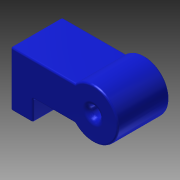
# Autodesk Inventor part: Lego Leg
Saved by Autodesk Inventor 2013 (Build 170138000, 138)
## iProperties
Created: 2013-09-06
Part Number: Lego Leg
Material: Generic
Document SubType Name: Modeling
Designer: 200395375
Density: 1 g/cm^3
Mass: 0.53052 g
Surface Area: 7.06359 cm^2
Volume: 0.53052 cm^3
Author: 200395375
Autodesk Inventor part; units mm, degrees
ref_plane "YZ Plane" through (0, 0, 0) normal (1, 0, 0) x (0, 1, 0)
ref_plane "XZ Plane" through (0, 0, 0) normal (0, 1, 0) x (-1, 0, 0)
ref_plane "XY Plane" through (0, 0, 0) normal (0, 0, 1) x (1, 0, 0)
sketch "Sketch1" plane through (0, 0, 0) normal (0, 1, 0) x (-1, 0, 0)
  line L0 (0, 0) -> (8.18, 0)
  line L1 (8.18, 0) -> (8.18, -7.83)
  line L2 (8.18, -7.83) -> (5.01, -7.83)
  line L3 (5.01, -7.83) -> (5.01, -4.86)
  line L4 (5.01, -4.86) -> (0, -4.86)
  line L5 (0, -4.86) -> (0, 0)
  dimension "d0" = 8.18
  dimension "d1" = 7.83
  dimension "d2" = 3.17
  dimension "d3" = 2.97
  constraints: 12 end point, 3 parallel, 2 perpendicular, 1 horizontal
  measures "d0" distance of L0.start L0.end
  measures "d1" distance of L0.end L1.end
  measures "d2" distance of L1.end L2.end
  measures "d3" distance of L2.end L3.end
extrude "Foot" add sketch "Sketch1" along normal blind 7.345
sketch "Sketch2" plane through (0, 7.345, 0) normal (0, 1, 0) x (1, 0, 0)
  line L0 (0, 0) -> (0, 4.86) projected
  circle A0 centre (3.54, 2.43) radius 3.54
  dimension "d6" = 7.08
  constraints: 1 centre point, 1 tangent
  measures "d6" diameter of A0
extrude "Leg" add sketch "Sketch2" against normal blind 7.345
sketch "Sketch3" plane through (0, 0, 0) normal (1, 0, 0) x (0, 0, -1)
  line L0 (2.43, 7.345) -> (2.43, 0) projected
  line L1 (0, 7.345) -> (2.43, 7.345) projected
  line L2 (0, 0) -> (0, 7.345) projected
  line L3 (2.43, 0) -> (0, 0) projected
extrude "Filling1" add sketch "Sketch3" along normal up to next
sketch "Sketch4" plane through (0, 0, -4.86) normal (1, 0, 0) x (0, 0, -1)
  line L0 (-2.43, 7.345) -> (-2.43, 0) projected
  line L1 (0, 0) -> (-2.43, 0) projected
  line L2 (0, 0) -> (0, 7.345) projected
  line L3 (-2.43, 7.345) -> (0, 7.345) projected
  point P0 (-4.86, 0)
extrude "Filling2" add sketch "Sketch4" along normal up to next
fillet "Fillet1" radius 0.25 17 edges at (-5.01, 3.6725, -7.83) (-5.01, 3.6725, -4.86) (-8.18, 7.345, -3.915) (-6.595, 7.345, -7.83) (-8.18, 3.6725, -7.83) (-5.01, 7.345, -6.345) (-2.0221, 7.345, -4.86) (-2.0221, 0, -4.86) (-5.01, 0, -6.345) (-6.595, 0, -7.83) (-3.6071, 7.345, 0) (-8.18, 3.6725, 0) (-8.18, 0, -3.915) (7.08, 7.345, -2.43) (7.08, 0, -2.43) (0.9658, 3.6725, -4.86) (-3.6071, 0, 0)
sketch "Sketch6" plane through (0, 0, 0) normal (0, -1, 0) x (1, 0, 0)
  arc A0 (1.2137, -4.7564) -> (1.2137, -4.7564) centre (3.54, -2.43) ccw projected
  circle A1 centre (3.54, -2.43) radius 0.75
  point P0 (1.0759, -0.25)
  point P1 (0, 0)
  dimension "d21" = 1.5
  constraints: 1 centre point, 1 coincident, 1 other
  measures "d21" diameter of A1
extrude "Hole" cut sketch "Sketch6" against normal blind 3 contours A1
fillet "Fillet5" radius 0.75 2 edges at (2.79, 3, -2.43) (2.79, 0, -2.43)
shell "Shell1" thickness 1.49 removed faces 0
sketch "Sketch7" plane through (-8.18, 0.25, -0.25) normal (-1, 0, 0) x (0, 0, 1)
  line L0 (0, 0) -> (-7.33, 0) projected
  line L1 (0, 6.845) -> (0, 0) projected
  line L2 (-7.33, 6.845) -> (0, 6.845) projected
  line L3 (-7.33, 0) -> (-7.33, 6.845) projected
  line L4 (-1.49, 1.49) -> (-5.84, 1.49)
  line L5 (-5.84, 1.49) -> (-5.84, 5.355)
  line L6 (-5.84, 5.355) -> (-1.49, 5.355)
  line L7 (-1.49, 5.355) -> (-1.49, 1.49)
  point P0 (0.25, -0.25)
  dimension "d26" = 1.49
  constraints: 8 end point, 3 other
  measures "d26" distance between parallel lines of L2 L6
extrude "Inside" cut sketch "Sketch7" against normal blind 1.49 contours L4 L5 L6 L7
fillet "Side" radius 0.25 8 edges at (-8.18, 5.605, -3.915) (-8.18, 3.6725, -1.74) (-8.18, 1.74, -3.915) (-8.18, 3.6725, -6.09) (-7.435, 5.605, -6.09) (-7.435, 5.605, -1.74) (-7.435, 1.74, -1.74) (-7.435, 1.74, -6.09)
body "Solid1"
